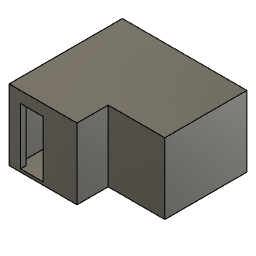
hab1 v7 (Autodesk Fusion 360 design; units mm, degrees)
Autodesk Fusion 360 part; units mm, degrees
sketch "Skizze1" plane through (0, 0, 0) normal (0, 1, 0) x (1, 0, 0)
  line L0 (0, 0) -> (0, 4000)
  line L1 (0, 4000) -> (4400, 4000)
  line L2 (4400, 4000) -> (4400, 1100)
  line L3 (4400, 1100) -> (2400, 1100)
  line L4 (2400, 1100) -> (2400, 0)
  line L5 (2400, 0) -> (0, 0)
  dimension "d1" = 4400
  dimension "d2" = 2900
  dimension "d3" = 4000
  dimension "d4" = 2400
  constraint coincident L0.start L5.end
  constraint vertical L0
  constraint perpendicular L0 L1
  constraint perpendicular L1 L2
  constraint perpendicular L2 L3
  constraint perpendicular L3 L4
  constraint perpendicular L0 L5
  measures "d1" distance of L0.end L1.end
  measures "d2" distance of L1.end L2.end
  measures "d3" distance of L0.start L0.end
  measures "d4" distance of L4.end L0.start
extrude "Extrusion1" add sketch "Skizze1" along normal blind 2400
sketch "Skizze2" plane through (0, 2400, 0) normal (0, 1, 0) x (-1, 0, 0)
  line L0 (-2400, 0) -> (-2400, -1100)
  line L1 (-2400, -1100) -> (-4400, -1100)
  line L2 (-4400, -1100) -> (-4400, -4000)
  line L3 (-4400, -4000) -> (0, -4000)
  line L4 (0, -4000) -> (0, 0)
  line L5 (0, 0) -> (-2400, 0)
  line L6 (-2200, -200) -> (-2200, -1200)
  line L7 (-2194.4735, -1300) -> (-4200, -1300)
  line L8 (-4200, -1300) -> (-4200, -3800)
  line L9 (-4200, -3800) -> (-200, -3800)
  line L10 (-200, -200) -> (-2200, -200)
  line L11 (-2194.4735, -1300) -> (-2000, -1300)
  line L12 (-2000, -1300) -> (-2000, -1200)
  line L13 (-2000, -1200) -> (-2200, -1200)
  line L14 (-200, -1300) -> (-1200, -1300)
  line L15 (-1200, -1300) -> (-1200, -1200)
  line L16 (-1200, -1200) -> (-200, -1200)
  line L17 (-200, -3800) -> (-200, -1300)
  line L18 (-200, -1200) -> (-200, -200)
  dimension "d9" = 100
  dimension "d10" = 800
  dimension "d11" = 100
  dimension "d12" = 200
  dimension "d13" = 200
  dimension "d14" = 200
  dimension "d15" = 200
  dimension "d16" = 200
  dimension "d17" = 200
  dimension "d18" = 200
  constraint perpendicular L6 L11
  constraint perpendicular L11 L12
  constraint perpendicular L6 L13
  constraint perpendicular L14 L17
  constraint perpendicular L14 L15
  constraint coincident L16.end L17
  constraint perpendicular L16 L17
  constraint parallel L0 L6
  constraint parallel L1 L7
  constraint parallel L2 L8
  constraint parallel L3 L9
  constraint parallel L4 L17
  constraint parallel L5 L10
  constraint collinear L17 L18
  constraint collinear L13 L16
  measures "d9" distance of L11.end L12.end
  measures "d10" distance of L12 L15
  measures "d11" distance of L14 L16
  measures "d12" distance of L12.end L6.end
  measures "d13" distance of L1 L7
  measures "d14" distance of L0 L6
  measures "d15" distance of L4 L18
  measures "d16" distance of L5 L10
  measures "d17" distance of L2 L8
  measures "d18" distance of L3 L9
extrude "Extrusion3" cut sketch "Skizze2" against normal blind 2300 contours L6 L7 L8 L9 L10 L11 L12 L13 L14 L15 L16 L17 L18
sketch "Skizze4" plane through (0, 0, 0) normal (0, 0, 1) x (1, 0, 0)
  line L0 (0, 0) -> (2400, 0)
  line L1 (2400, 0) -> (2400, 2400)
  line L2 (2400, 2400) -> (0, 2400)
  line L3 (0, 2400) -> (0, 0)
  line L4 (400, 100) -> (1200, 100)
  line L5 (1200, 100) -> (1200, 2100)
  line L6 (1200, 2100) -> (400, 2100)
  line L7 (400, 2100) -> (400, 100)
  dimension "d23" = 100
  dimension "d24" = 800
  dimension "d25" = 2000
  dimension "d26" = 400
  constraint horizontal L4
  constraint vertical L5
  constraint horizontal L6
  constraint vertical L7
  measures "d23" distance of L0 L4
  measures "d24" distance of L5 L7
  measures "d25" distance of L4.end L5.end
  measures "d26" distance of L3 L7
extrude "Extrusion4" cut sketch "Skizze4" against normal up to surface (1200 mm away) contours L4 L5 L6 L7
sketch "Skizze5" plane through (2000, 0, 0) normal (-1, 0, 0) x (0, 0, 1)
  line L0 (-1200, 2400) -> (-1300, 2400)
  line L1 (-1300, 2400) -> (-1300, 100)
  line L2 (-1300, 100) -> (-1200, 100)
  line L3 (-1200, 100) -> (-1200, 2400)
  line L4 (-1300, 2400) -> (-1200, 2400)
  line L5 (-1200, 2400) -> (-1200, 2100)
  line L6 (-1200, 2100) -> (-1300, 2100)
  line L7 (-1300, 2100) -> (-1300, 2400)
  dimension "d29" = 300
  constraint horizontal L4
  constraint vertical L5
  constraint horizontal L6
  constraint vertical L7
  constraint coincident L3 L5.end
  constraint coincident L0.end L1.start
  measures "d29" distance of L0.start L5.end
extrude "Extrusion5" add sketch "Skizze5" along normal up to surface (800 mm away) contours L0 L1 L3 L4 L5 L6 L7
sketch "Skizze6" plane through (0, 2400, 0) normal (0, 1, 0) x (-1, 0, 0)
  line L0 (-4200, -1300) -> (-200, -1300)
  line L1 (-200, -1300) -> (-200, -3800)
  line L2 (-200, -3800) -> (-4200, -3800)
  line L3 (-4200, -3800) -> (-4200, -1300)
  line L4 (-200, -1200) -> (-2200, -1200)
  line L5 (-2200, -1200) -> (-2200, -200)
  line L6 (-2200, -200) -> (-200, -200)
  line L7 (-200, -200) -> (-200, -1200)
  line L8 (-2400, 0) -> (-2400, -1100)
  line L9 (-2400, -1100) -> (-4400, -1100)
  line L10 (-4400, -1100) -> (-4400, -4000)
  line L11 (-4400, -4000) -> (0, -4000)
  line L12 (0, -4000) -> (0, 0)
  line L13 (0, 0) -> (-2400, 0)
extrude "Extrusion6" add sketch "Skizze6" along normal blind 100 contours L0 L1 L2 L3 | L4 L5 L6 L7 | L8 L9 L10 L11 L12 L13
sketch "Skizze7" plane through (0, 0, -4000) normal (0, 0, -1) x (-1, 0, 0)
  line L0 (-4400, 0) -> (0, 0)
  line L1 (0, 0) -> (0, 2500)
  line L2 (0, 2500) -> (-4400, 2500)
  line L3 (-4400, 2500) -> (-4400, 0)
  line L4 (-2514.864, 1700) -> (-1914.864, 1700)
  line L5 (-1914.864, 1700) -> (-1914.864, 1000)
  line L6 (-1914.864, 1000) -> (-2514.864, 1000)
  line L7 (-2514.864, 1000) -> (-2514.864, 1700)
  line L8 (-200, 100) -> (-4200, 100)
  dimension "d34" = 600
  dimension "d35" = 700
  dimension "d36" = 900
  constraint horizontal L4
  constraint vertical L5
  constraint horizontal L6
  constraint vertical L7
  measures "d34" distance of L4.start L4.end
  measures "d35" distance of L4.start L6.end
  measures "d36" distance of L6 L8
extrude "Extrusion7" cut sketch "Skizze7" against normal blind 300 contours L4 L5 L6 L7
extrude "Extrusion2" [rolled back] along distance 2200 taper angle 0
